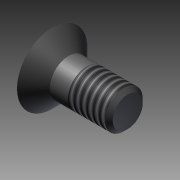
# Autodesk Inventor part: FB3-6s
Saved by Autodesk Inventor 2011 SP1 (Build 150282100, 282)
## iProperties
Created: 2015-02-01
Part Number: FB3-6s
Catalog Web Link: www.cadenas.de
Description: FB-11-Hexagon Socket Head Cap Screws-11
Vendor: MISUMI
Document SubType Name: Modeling
Designer: psAdmin
Manufacturer: MISUMI
Mass: 0.0462916 g
Surface Area: 1.08321 cm^2
Volume: 0.0462916 cm^3
Density: 1 g/cm^3
Category: PARTsolutions
Company: MISUMI
Title: FB3-6s
Author: Cadenas PARTsolutions
Comments: Hexagon Socket Head Cap Screws-11
PSOL_IDENT_0: {\\10.0.0.236\data_v8\23d-libs\misumi\metric\39_accessories_for_al_extrusions\fb11.prj},155 {VTYP=3D
PSOL_IDENT_1: },{NB=FB3-6s},{LINA=FB3-6s},{NN=FB-11},{DATE=17.11.2014 05:30:42},{GEOMDATE=17.02.2014 00:00:00},{VE
PSOL_IDENT_2: RSION=},{LINEID=150},{LINESUBID=-1},{WBVAR=L}  {NB=FB3-6s},{LINA=FB3-6s},{KT=DUMMY},{PN=FB3-6s},{MAT=
PSOL_IDENT_3: 4137 Steel},{HARD=32~38HRC},{M=3},{L=6},{LL=Full Thread},{L1=22},{TYPE=FB},{L0=6,8,10},{NDM=3},{KDM=
PSOL_IDENT_4: 1.156995},{MP=3x1.5},{P=1.5},{A=20},{E=5.5},{B=6.0}
SUPPLIER: MISUMI
ARTICLENO: FB3-6s
BOMINFO: FB3-6s
CREATOR: CADENAS GmbH
Autodesk Inventor part; units mm, degrees
sketch "Sketch_8" plane through (0, 0, 0) normal (0, 0, 1) x (1, 0, 0)
  line L0 (6, 0) -> (0, 0)
  line L1 (0, 0) -> (0, 2.8)
  line L2 (0, 2.8) -> (1.3, 1.5)
  line L3 (1.3, 1.5) -> (5.6935, 1.5)
  line L4 (5.6935, 1.5) -> (6, 1.1935)
  line L5 (6, 1.1935) -> (6, 0)
  line L6 (6, 0) -> (0, 0)
  constraints: 14 end point
revolve "Revolution1" add sketch "Sketch_8" angle 360 about axis through (6, 0, 0) along (1, 0, 0)
thread "Thread1" size "M3x0.5" class "6g" standard "ISO Metric profile" length 3.25 offset 1.45
sketch "Sketch_9" plane through (0, 0, 0) normal (0, 1, 0) x (-1, 0, 0)
  line L0 (-1.4215, 0) -> (0, 0)
  line L1 (0, 0) -> (0, -1.2)
  line L2 (0, -1.2) -> (-1.1, -1.2)
  line L3 (-1.1, -1.2) -> (-1.4215, 0)
  line L4 (-1.4215, 0) -> (0, 0)
  constraints: 10 end point
revolve "Revolution2" cut sketch "Sketch_9" angle 360 about axis through (1.4215, 0, 0) along (1, 0, 0)
sketch "Sketch_10" plane through (0, 0, 0) normal (1, 0, 0) x (0, 1, 0)
  line L0 (0.6928, 1.2) -> (-0.6928, 1.2)
  line L1 (-0.6928, 1.2) -> (-1.3856, 0)
  line L2 (-1.3856, 0) -> (-0.6928, -1.2)
  line L3 (-0.6928, -1.2) -> (0.6928, -1.2)
  line L4 (0.6928, -1.2) -> (1.3856, 0)
  line L5 (1.3856, 0) -> (0.6928, 1.2)
  constraints: 12 end point
extrude "Extrusion1" cut sketch "Sketch_10" along normal blind 1.1
ref_plane "screw_XY" through (5.5, 0, 0) normal (1, 0, 0) x (0, 0, -1)
ref_plane "screw_YZ" through (5.5, 0, 0) normal (0, 0, -1) x (0, 1, 0)
ref_plane "screw_ZX" through (5.5, 0, 0) normal (0, 1, 0) x (1, 0, 0)
ref_plane "to_nut_XY" through (6, 0, 0) normal (1, 0, 0) x (0, 0, -1)
ref_plane "to_nut_YZ" through (6, 0, 0) normal (0, 0, -1) x (0, 1, 0)
ref_plane "to_nut_ZX" through (6, 0, 0) normal (0, 1, 0) x (1, 0, 0)
ref_plane "xx_XY" through (0.8, 0, 0) normal (1, 0, 0) x (0, 0, -1)
ref_plane "xx_YZ" through (0.8, 0, 0) normal (0, 0, -1) x (0, 1, 0)
ref_plane "xx_ZX" through (0.8, 0, 0) normal (0, 1, 0) x (1, 0, 0)
body "Solid1"
